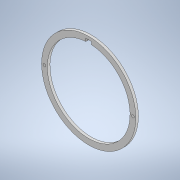
# Autodesk Inventor part: Montage_Ring_Vorne
Saved by Autodesk Inventor 2022.2 (Build 262287010, 287A)
## iProperties
Created: 2024-01-10
Part Number: Montage_Ring_Vorne
Material: Generisch
Document SubType Name: Modeling
Designer: ppovolni
Density: 1 g/cm^3
Appearance: Vorgabe
Author: ppovolni
Autodesk Inventor part; units mm, degrees
ref_plane "YZ Plane" through (0, 0, 0) normal (1, 0, 0) x (0, 1, 0)
ref_plane "XZ Plane" through (0, 0, 0) normal (0, 1, 0) x (-1, 0, 0)
ref_plane "XY Plane" through (0, 0, 0) normal (0, 0, 1) x (1, 0, 0)
sketch "Skizze1" plane through (0, 0, 0) normal (0, 0, 1) x (1, 0, 0)
  circle A0 centre (0, 0) radius 80.1 construction
  circle A1 centre (0, 0) radius 93.8 construction
  circle A2 centre (0, 0) radius 80.6
  circle A3 centre (0, 0) radius 91.8
  arc A4 (5.5, 85.9242) -> (-5.5, 85.9242) centre (0, 0) ccw
  line L0 (-5.5, 85.9242) -> (-5.5, 80.4121)
  line L1 (5.5, 85.9242) -> (5.5, 80.4121)
  point P0 (0, 86.1)
  dimension "d0" = 187.6
  dimension "d1" = 160.2
  dimension "d2" = 2
  dimension "d3" = 0.5
  dimension "d6" = 6
  dimension "d7" = 11
  constraints: 5 centre point, 5 coincident, 5 point on circle, 4 end point, 2 vertical, 1 vertical alignment
  measures "d0" diameter of A1
  measures "d1" diameter of A0
  measures "d2" radial gap between concentric circles of A1 A3
  measures "d3" radial gap between concentric circles of A0 A2
  measures "d6" radial gap between concentric circles of A0 A4
  measures "d7" distance of L1.start L0.start
extrude "Extrusion1" add sketch "Skizze1" along normal blind 5
sketch "Skizze2" plane through (0, 0, 5) normal (0, 0, 1) x (1, 0, 0)
  circle A0 centre (-86.2, 0) radius 2.6
  circle A1 centre (86.2, 0) radius 2.6
  line L0 (-86.2, 0) -> (86.2, 0) construction
  arc A2 (-5.5, 80.4121) -> (5.5, 80.4121) centre (0, 0) ccw construction
  point P0 (-80.6, 0)
  point P1 (80.6, 0)
  dimension "d8" = 5.2
  dimension "d9" = 5.6
  dimension "d10" = 5.6
  constraints: 2 centre point, 2 end point, 2 point on circle, 2 point on line, 1 equal radius, 1 horizontal, 1 midpoint
  measures "d8" diameter of A0
  measures "d9" distance of L0.start point (-80.6, 0)
  measures "d10" distance of L0.end point (80.6, 0)
extrude "Extrusion2" cut sketch "Skizze2" against normal blind 5
